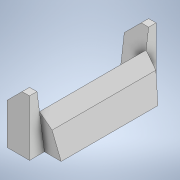
# Autodesk Inventor part: inside-join
Saved by Autodesk Inventor 2021 (Build 250183000, 183)
## iProperties
Created: 2020-12-08
Part Number: inside-join
Material: Generic
Document SubType Name: Modeling
Designer: Luke Kamols
Density: 1 g/cm^3
Appearance: Default
Author: Luke Kamols
Autodesk Inventor part; units mm, degrees
ref_plane "YZ Plane" through (0, 0, 0) normal (1, 0, 0) x (0, 1, 0)
ref_plane "XZ Plane" through (0, 0, 0) normal (0, 1, 0) x (-1, 0, 0)
ref_plane "XY Plane" through (0, 0, 0) normal (0, 0, 1) x (1, 0, 0)
sketch "Sketch1" plane through (0, 0, 0) normal (0, 0, 1) x (1, 0, 0)
  line L0 (0, 10) -> (3, 7)
  line L1 (0, 10) -> (4.2426, 10) construction
  line L2 (0, 10) -> (-4.2426, 10) construction
  line L3 (4.5, 0) -> (3, 7)
  line L4 (0, 0) -> (4.5, 0)
  line L5 (0, 10) -> (-3, 7)
  line L6 (0, 10) -> (-4.2426, 10) construction
  line L7 (-4.5, 0) -> (-3, 7)
  line L8 (0, 0) -> (-4.5, 0)
  dimension "d2" = 45
  constraints: 18 end point, 2 horizontal, 1 equal length
  measures "d2" angle of L0 L1
extrude "Extrusion1" add sketch "Sketch1" along normal blind 26
sketch "Sketch2" plane through (0, 0, 26) normal (0, 0, 1) x (1, 0, 0)
  line L0 (0, 0) -> (0, 15)
  line L1 (0, 15) -> (-2, 15)
  line L2 (0, 0) -> (-6, 0)
  line L3 (-4.5, 0) -> (4.5, 0) projected
  line L4 (-6, 0) -> (-6, 11)
  line L5 (-6, 11) -> (-2, 15)
  dimension "d6" = 15
  dimension "d7" = 2
  dimension "d8" = 6
  dimension "d9" = 11
  constraints: 10 end point, 2 perpendicular, 1 collinear, 1 vertical
  measures "d6" distance of L0.start L0.end
  measures "d7" distance of L0.end L1.end
  measures "d8" distance of L0.start L2.end
  measures "d9" distance of L2.end L4.end
extrude "Extrusion2" add sketch "Sketch2" along normal blind 4
sketch "Sketch3" plane through (0, 10, 26) normal (1, 0, 0) x (0, 0, -1)
  line L0 (0, -3) -> (0, -10) projected
  line L1 (0, -10) -> (-2, 5)
  line L2 (0, 5) -> (-4, 5) projected
  line L3 (0, 0) -> (0, 5) projected
  line L4 (-2, 5) -> (0, 5)
  line L5 (26, -10) -> (0, -10) projected
  line L6 (0, 5) -> (0, -10)
  constraints: 6 end point, 1 horizontal, 1 midpoint, 1 perpendicular
extrude "Extrusion3" cut sketch "Sketch3" against normal blind 8.7625
sketch "Sketch4" plane through (0, 0, 26) normal (0, 0, 1) x (1, 0, 0)
  line L0 (4.5, 0) -> (3, 7) projected
  line L1 (4.5, 0) -> (3, 7)
  line L2 (3, 7) -> (0, 10) projected
  line L3 (3, 7) -> (0, 10)
  line L4 (0, 10) -> (-3, 7) projected
  line L5 (0, 10) -> (-3, 7)
  line L6 (-3, 7) -> (-4.5, 0) projected
  line L7 (-3, 7) -> (-4.5, 0)
  line L8 (0, 0) -> (4.5, 0) projected
  line L9 (-4.5, 0) -> (4.5, 0)
  constraints: 10 end point, 5 collinear
extrude "Extrusion4" add sketch "Sketch4" against normal up to surface surface through (0, 0, 26) normal (0, -0.1321637, 0.9912279)
sketch "Sketch5" plane through (0, 0, 0) normal (0, 0, -1) x (-1, 0, 0)
  line L0 (0, 0) -> (6, 0)
  line L1 (4.5, 0) -> (-4.5, 0) projected
  line L2 (0, 10) -> (0, 15) projected
  line L3 (0, 0) -> (0, 15)
  line L4 (0, 15) -> (2, 15) projected
  line L5 (0, 15) -> (2, 15)
  line L6 (6, 0) -> (0, 0) projected
  line L7 (6, 11) -> (6, 0) projected
  line L8 (6, 0) -> (6, 11)
  line L9 (2, 15) -> (6, 11) projected
  line L10 (6, 11) -> (2, 15)
  dimension "d18" = 11
  constraints: 10 end point, 3 collinear, 2 vertical
  measures "d18" distance of L0.end L7.start
extrude "Extrusion5" add sketch "Sketch5" along normal blind 4
sketch "Sketch6" plane through (0, 10, 0) normal (1, 0, 0) x (0, 0, -1)
  line L0 (0, -10) -> (2, 5)
  line L1 (0, 5) -> (4, 5) projected
  line L2 (0, 5) -> (4, 5) projected
  line L3 (2, 5) -> (0, 5)
  line L4 (0, -10) -> (0, 0) projected
  line L5 (0, 5) -> (0, -10)
  constraints: 6 end point, 1 collinear, 1 horizontal, 1 midpoint
extrude "Extrusion6" cut sketch "Sketch6" against normal blind 10.35
sketch "Sketch7" plane through (0, 0, 0) normal (0, 0, -1) x (-1, 0, 0)
  line L0 (0, 0) -> (-4.5, 0) projected
  line L1 (-4.5, 0) -> (-3, 7) projected
  line L2 (-4.5, 0) -> (-3, 7)
  line L3 (0, 10) -> (3, 7) projected
  line L4 (-3, 7) -> (0, 10)
  line L5 (3, 7) -> (4.5, 0) projected
  line L6 (0, 10) -> (3, 7)
  line L7 (3, 7) -> (4.5, 0)
  line L8 (4.5, 0) -> (-4.5, 0)
  constraints: 10 end point, 2 collinear, 2 perpendicular, 1 horizontal
extrude "Extrusion7" add sketch "Sketch7" against normal up to surface surface through (0, 15, -2) normal (0, -0.1321637, -0.9912279)
body "Solid1"
